Autodesk Inventor part; units mm, degrees
(part 2 of 2)
sketch "Sketch75" plane through (47.5, -21.3496, 62.3406) normal (0, 0.5735764, 0.819152) x (1, 0, 0)
  line L0 (-6.516, 66.3057) -> (-44.6738, 66.3057) construction
  line L1 (-44.6738, 66.3057) -> (-44.6738, 71.3022) construction
  line L2 (-44.6738, 71.3022) -> (-6.516, 71.3022) construction
  line L3 (-6.516, 71.3022) -> (-6.516, 66.3057) construction
  line L4 (-3.768, 77.8286) -> (-3.768, -61.6175) projected
  spline S0 degree 2 poles (-9.2281, 67.8964) (-9.2281, 68.3138) (-8.8897, 68.9857) (-8.6056, 69.1734) knots 0 0 0 1 2 2 2
  spline S1 degree 2 poles (-8.6056, 69.1734) (-8.3735, 69.3191) (-7.8967, 69.4179) (-7.5262, 69.4179) knots 0 0 0 1 2 2 2
  line L5 (-7.5262, 69.4179) -> (-6.8248, 69.4179)
  line L6 (-6.8248, 69.4179) -> (-6.8248, 66.3699)
  line L7 (-6.8248, 66.3699) -> (-7.5188, 66.3699)
  spline S2 degree 2 poles (-7.5188, 66.3699) (-7.9486, 66.3699) (-8.4377, 66.4984) (-8.6106, 66.612) knots 0 0 0 1 2 2 2
  spline S3 degree 2 poles (-8.6106, 66.612) (-8.9045, 66.8071) (-9.2281, 67.4518) (-9.2281, 67.8964) knots 0 0 0 1 2 2 2
  spline S4 degree 2 poles (-8.8057, 67.8915) (-8.8057, 67.5407) (-8.5735, 67.0443) (-8.3438, 66.9035) knots 0 0 0 1 2 2 2
  spline S5 degree 2 poles (-8.3438, 66.9035) (-8.1808, 66.8071) (-7.8128, 66.7207) (-7.5386, 66.7207) knots 0 0 0 1 2 2 2
  line L8 (-7.5386, 66.7207) -> (-7.2298, 66.7207)
  line L9 (-7.2298, 66.7207) -> (-7.2298, 69.0672)
  line L10 (-7.2298, 69.0672) -> (-7.5386, 69.0672)
  spline S6 degree 2 poles (-7.5386, 69.0672) (-7.8078, 69.0672) (-8.2154, 68.9808) (-8.3809, 68.8647) knots 0 0 0 1 2 2 2
  spline S7 degree 2 poles (-8.3809, 68.8647) (-8.5933, 68.7214) (-8.8057, 68.2472) (-8.8057, 67.8915) knots 0 0 0 1 2 2 2
  spline S8 degree 2 poles (-10.7323, 69.4822) (-10.4631, 69.4822) (-10.0629, 69.3414) (-9.9222, 69.2006) knots 0 0 0 1 2 2 2
  spline S9 degree 2 poles (-9.9222, 69.2006) (-9.7616, 69.0425) (-9.6307, 68.5979) (-9.6307, 68.2719) knots 0 0 0 1 2 2 2
  line L11 (-9.6307, 68.2719) -> (-9.6307, 66.3699)
  line L12 (-9.6307, 66.3699) -> (-10.0358, 66.3699)
  line L13 (-10.0358, 66.3699) -> (-10.0358, 68.2719)
  spline S10 degree 2 poles (-10.0358, 68.2719) (-10.0358, 68.4843) (-10.0901, 68.7708) (-10.1667, 68.8869) knots 0 0 0 1 2 2 2
  spline S11 degree 2 poles (-10.1667, 68.8869) (-10.2482, 69.0104) (-10.5298, 69.1364) (-10.7323, 69.1364) knots 0 0 0 1 2 2 2
  spline S12 degree 2 poles (-10.7323, 69.1364) (-10.9225, 69.1364) (-11.2189, 69.0104) (-11.3004, 68.8869) knots 0 0 0 1 2 2 2
  spline S13 degree 2 poles (-11.3004, 68.8869) (-11.377, 68.7708) (-11.4313, 68.4867) (-11.4313, 68.2817) knots 0 0 0 1 2 2 2
  line L14 (-11.4313, 68.2817) -> (-11.4313, 66.3699)
  line L15 (-11.4313, 66.3699) -> (-11.8364, 66.3699)
  line L16 (-11.8364, 66.3699) -> (-11.8364, 68.2719)
  spline S14 degree 2 poles (-11.8364, 68.2719) (-11.8364, 68.5905) (-11.708, 69.045) (-11.545, 69.2006) knots 0 0 0 1 2 2 2
  spline S15 degree 2 poles (-11.545, 69.2006) (-11.3992, 69.3438) (-11.0139, 69.4822) (-10.7323, 69.4822) knots 0 0 0 1 2 2 2
  line L17 (-12.0884, 69.4179) -> (-13.1159, 66.3699)
  line L18 (-13.1159, 66.3699) -> (-13.6148, 66.3699)
  line L19 (-13.6148, 66.3699) -> (-14.6424, 69.4179)
  line L20 (-14.6424, 69.4179) -> (-14.215, 69.4179)
  line L21 (-14.215, 69.4179) -> (-13.9384, 68.5658)
  line L22 (-13.9384, 68.5658) -> (-12.775, 68.5658)
  line L23 (-12.775, 68.5658) -> (-12.4984, 69.4179)
  line L24 (-12.4984, 69.4179) -> (-12.0884, 69.4179)
  line L25 (-13.8272, 68.22) -> (-13.3555, 66.7849)
  line L26 (-13.3555, 66.7849) -> (-12.8862, 68.22)
  line L27 (-12.8862, 68.22) -> (-13.8272, 68.22)
  line L28 (-16.6974, 69.4179) -> (-14.9313, 69.4179)
  line L29 (-14.9313, 69.4179) -> (-14.9313, 66.3699)
  line L30 (-14.9313, 66.3699) -> (-15.3364, 66.3699)
  line L31 (-15.3364, 66.3699) -> (-15.3364, 69.0573)
  line L32 (-15.3364, 69.0573) -> (-16.6974, 69.0573)
  line L33 (-16.6974, 69.0573) -> (-16.6974, 69.4179)
  line L34 (-20.5358, 66.3699) -> (-19.4861, 69.4179)
  line L35 (-19.4861, 69.4179) -> (-19.0489, 69.4179)
  line L36 (-19.0489, 69.4179) -> (-17.9991, 66.3699)
  line L37 (-17.9991, 66.3699) -> (-18.4338, 66.3699)
  line L38 (-18.4338, 66.3699) -> (-19.2786, 68.9017)
  line L39 (-19.2786, 68.9017) -> (-20.1233, 66.3699)
  line L40 (-20.1233, 66.3699) -> (-20.5358, 66.3699)
  line L41 (-21.8894, 69.4179) -> (-20.7087, 69.4179)
  line L42 (-20.7087, 69.4179) -> (-20.7087, 69.1067)
  line L43 (-20.7087, 69.1067) -> (-21.0965, 69.1067)
  line L44 (-21.0965, 69.1067) -> (-21.0965, 66.6812)
  line L45 (-21.0965, 66.6812) -> (-20.7087, 66.6812)
  line L46 (-20.7087, 66.6812) -> (-20.7087, 66.3699)
  line L47 (-20.7087, 66.3699) -> (-21.8894, 66.3699)
  line L48 (-21.8894, 66.3699) -> (-21.8894, 66.6812)
  line L49 (-21.8894, 66.6812) -> (-21.5016, 66.6812)
  line L50 (-21.5016, 66.6812) -> (-21.5016, 69.1067)
  line L51 (-21.5016, 69.1067) -> (-21.8894, 69.1067)
  line L52 (-21.8894, 69.1067) -> (-21.8894, 69.4179)
  spline S16 degree 2 poles (-23.2405, 69.4723) (-22.9095, 69.4723) (-22.4451, 69.334) (-22.2401, 69.2352) knots 0 0 0 1 2 2 2
  line L53 (-22.2401, 69.2352) -> (-22.2401, 68.7263)
  line L54 (-22.2401, 68.7263) -> (-22.2698, 68.7263)
  spline S17 degree 2 poles (-22.2698, 68.7263) (-22.4698, 68.9141) (-22.9762, 69.1215) (-23.2108, 69.1215) knots 0 0 0 1 2 2 2
  spline S18 degree 2 poles (-23.2108, 69.1215) (-23.5468, 69.1215) (-23.8901, 68.8424) (-23.8901, 68.6127) knots 0 0 0 1 2 2 2
  spline S19 degree 2 poles (-23.8901, 68.6127) (-23.8901, 68.4299) (-23.7098, 68.2027) (-23.5147, 68.1459) knots 0 0 0 1 2 2 2
  spline S20 degree 2 poles (-23.5147, 68.1459) (-23.3739, 68.1064) (-23.1392, 68.052) (-22.9638, 68.0076) knots 0 0 0 1 2 2 2
  spline S21 degree 2 poles (-22.9638, 68.0076) (-22.8058, 67.9656) (-22.5563, 67.8396) (-22.46, 67.7383) knots 0 0 0 1 2 2 2
  spline S22 degree 2 poles (-22.46, 67.7383) (-22.3661, 67.6371) (-22.2624, 67.3654) (-22.2624, 67.1875) knots 0 0 0 1 2 2 2
  spline S23 degree 2 poles (-22.2624, 67.1875) (-22.2624, 66.817) (-22.8403, 66.3156) (-23.2874, 66.3156) knots 0 0 0 1 2 2 2
  spline S24 degree 2 poles (-23.2874, 66.3156) (-23.5443, 66.3156) (-23.9988, 66.4169) (-24.1939, 66.5132) knots 0 0 0 1 2 2 2
  line L55 (-24.1939, 66.5132) -> (-24.1939, 66.9973)
  line L56 (-24.1939, 66.9973) -> (-24.1643, 66.9973)
  spline S25 degree 2 poles (-24.1643, 66.9973) (-24.0185, 66.8639) (-23.5641, 66.6663) (-23.3146, 66.6663) knots 0 0 0 1 2 2 2
  spline S26 degree 2 poles (-23.3146, 66.6663) (-23.033, 66.6663) (-22.6847, 66.9306) (-22.6847, 67.1455) knots 0 0 0 1 2 2 2
  spline S27 degree 2 poles (-22.6847, 67.1455) (-22.6847, 67.3382) (-22.8897, 67.5679) (-23.0824, 67.6198) knots 0 0 0 1 2 2 2
  spline S28 degree 2 poles (-23.0824, 67.6198) (-23.2108, 67.6544) (-23.5838, 67.7433) (-23.7073, 67.7803) knots 0 0 0 1 2 2 2
  spline S29 degree 2 poles (-23.7073, 67.7803) (-24.021, 67.8767) (-24.3125, 68.2644) (-24.3125, 68.5485) knots 0 0 0 1 2 2 2
  spline S30 degree 2 poles (-24.3125, 68.5485) (-24.3125, 68.7288) (-24.1667, 69.0746) (-24.0358, 69.1956) knots 0 0 0 1 2 2 2
  spline S31 degree 2 poles (-24.0358, 69.1956) (-23.8901, 69.329) (-23.5196, 69.4723) (-23.2405, 69.4723) knots 0 0 0 1 2 2 2
  line L57 (-25.7871, 69.4179) -> (-24.6064, 69.4179)
  line L58 (-24.6064, 69.4179) -> (-24.6064, 69.1067)
  line L59 (-24.6064, 69.1067) -> (-24.9942, 69.1067)
  line L60 (-24.9942, 69.1067) -> (-24.9942, 66.6812)
  line L61 (-24.9942, 66.6812) -> (-24.6064, 66.6812)
  line L62 (-24.6064, 66.6812) -> (-24.6064, 66.3699)
  line L63 (-24.6064, 66.3699) -> (-25.7871, 66.3699)
  line L64 (-25.7871, 66.3699) -> (-25.7871, 66.6812)
  line L65 (-25.7871, 66.6812) -> (-25.3993, 66.6812)
  line L66 (-25.3993, 66.6812) -> (-25.3993, 69.1067)
  line L67 (-25.3993, 69.1067) -> (-25.7871, 69.1067)
  line L68 (-25.7871, 69.1067) -> (-25.7871, 69.4179)
  spline S32 degree 2 poles (-28.4448, 66.7182) (-28.6177, 66.9208) (-28.8104, 67.5136) (-28.8104, 67.8939) knots 0 0 0 1 2 2 2
  spline S33 degree 2 poles (-28.8104, 67.8939) (-28.8104, 68.2644) (-28.6226, 68.8647) (-28.4448, 69.0672) knots 0 0 0 1 2 2 2
  spline S34 degree 2 poles (-28.4448, 69.0672) (-28.2571, 69.2796) (-27.7606, 69.4822) (-27.4617, 69.4822) knots 0 0 0 1 2 2 2
  spline S35 degree 2 poles (-27.4617, 69.4822) (-27.153, 69.4822) (-26.659, 69.2722) (-26.4787, 69.0672) knots 0 0 0 1 2 2 2
  spline S36 degree 2 poles (-26.4787, 69.0672) (-26.3033, 68.8647) (-26.1156, 68.2694) (-26.1156, 67.8939) knots 0 0 0 1 2 2 2
  spline S37 degree 2 poles (-26.1156, 67.8939) (-26.1156, 67.5111) (-26.3058, 66.9282) (-26.4811, 66.7182) knots 0 0 0 1 2 2 2
  spline S38 degree 2 poles (-26.4811, 66.7182) (-26.659, 66.5157) (-27.1555, 66.3057) (-27.4617, 66.3057) knots 0 0 0 1 2 2 2
  spline S39 degree 2 poles (-27.4617, 66.3057) (-27.773, 66.3057) (-28.2719, 66.5231) (-28.4448, 66.7182) knots 0 0 0 1 2 2 2
  spline S40 degree 2 poles (-28.388, 67.8939) (-28.388, 67.5926) (-28.2571, 67.1258) (-28.1385, 66.9726) knots 0 0 0 1 2 2 2
  spline S41 degree 2 poles (-28.1385, 66.9726) (-28.0175, 66.8145) (-27.6766, 66.6565) (-27.4642, 66.6565) knots 0 0 0 1 2 2 2
  spline S42 degree 2 poles (-27.4642, 66.6565) (-27.2444, 66.6565) (-26.9134, 66.8096) (-26.7874, 66.9726) knots 0 0 0 1 2 2 2
  spline S43 degree 2 poles (-26.7874, 66.9726) (-26.6664, 67.1282) (-26.538, 67.5975) (-26.538, 67.8939) knots 0 0 0 1 2 2 2
  spline S44 degree 2 poles (-26.538, 67.8939) (-26.538, 68.4942) (-27.0418, 69.1314) (-27.4642, 69.1314) knots 0 0 0 1 2 2 2
  spline S45 degree 2 poles (-27.4642, 69.1314) (-27.8866, 69.1314) (-28.388, 68.4942) (-28.388, 67.8939) knots 0 0 0 1 2 2 2
  line L69 (-31.436, 69.4179) -> (-30.9815, 69.4179)
  line L70 (-30.9815, 69.4179) -> (-29.6329, 66.7898)
  line L71 (-29.6329, 66.7898) -> (-29.6329, 69.4179)
  line L72 (-29.6329, 69.4179) -> (-29.255, 69.4179)
  line L73 (-29.255, 69.4179) -> (-29.255, 66.3699)
  line L74 (-29.255, 66.3699) -> (-29.8305, 66.3699)
  line L75 (-29.8305, 66.3699) -> (-31.0581, 68.7832)
  line L76 (-31.0581, 68.7832) -> (-31.0581, 66.3699)
  line L77 (-31.0581, 66.3699) -> (-31.436, 66.3699)
  line L78 (-31.436, 66.3699) -> (-31.436, 69.4179)
  line L79 (-35.1287, 69.4179) -> (-33.3626, 69.4179)
  line L80 (-33.3626, 69.4179) -> (-33.3626, 66.3699)
  line L81 (-33.3626, 66.3699) -> (-33.7677, 66.3699)
  line L82 (-33.7677, 66.3699) -> (-33.7677, 69.0573)
  line L83 (-33.7677, 69.0573) -> (-35.1287, 69.0573)
  line L84 (-35.1287, 69.0573) -> (-35.1287, 69.4179)
  line L85 (-36.5094, 69.4179) -> (-35.3287, 69.4179)
  line L86 (-35.3287, 69.4179) -> (-35.3287, 69.1067)
  line L87 (-35.3287, 69.1067) -> (-35.7165, 69.1067)
  line L88 (-35.7165, 69.1067) -> (-35.7165, 66.6812)
  line L89 (-35.7165, 66.6812) -> (-35.3287, 66.6812)
  line L90 (-35.3287, 66.6812) -> (-35.3287, 66.3699)
  line L91 (-35.3287, 66.3699) -> (-36.5094, 66.3699)
  line L92 (-36.5094, 66.3699) -> (-36.5094, 66.6812)
  line L93 (-36.5094, 66.6812) -> (-36.1216, 66.6812)
  line L94 (-36.1216, 66.6812) -> (-36.1216, 69.1067)
  line L95 (-36.1216, 69.1067) -> (-36.5094, 69.1067)
  line L96 (-36.5094, 69.1067) -> (-36.5094, 69.4179)
  spline S46 degree 2 poles (-39.4141, 67.8964) (-39.4141, 68.3138) (-39.0758, 68.9857) (-38.7917, 69.1734) knots 0 0 0 1 2 2 2
  spline S47 degree 2 poles (-38.7917, 69.1734) (-38.5595, 69.3191) (-38.0828, 69.4179) (-37.7123, 69.4179) knots 0 0 0 1 2 2 2
  line L97 (-37.7123, 69.4179) -> (-37.0108, 69.4179)
  line L98 (-37.0108, 69.4179) -> (-37.0108, 66.3699)
  line L99 (-37.0108, 66.3699) -> (-37.7049, 66.3699)
  spline S48 degree 2 poles (-37.7049, 66.3699) (-38.1347, 66.3699) (-38.6237, 66.4984) (-38.7966, 66.612) knots 0 0 0 1 2 2 2
  spline S49 degree 2 poles (-38.7966, 66.612) (-39.0906, 66.8071) (-39.4141, 67.4518) (-39.4141, 67.8964) knots 0 0 0 1 2 2 2
  spline S50 degree 2 poles (-38.9918, 67.8915) (-38.9918, 67.5407) (-38.7596, 67.0443) (-38.5299, 66.9035) knots 0 0 0 1 2 2 2
  spline S51 degree 2 poles (-38.5299, 66.9035) (-38.3669, 66.8071) (-37.9988, 66.7207) (-37.7247, 66.7207) knots 0 0 0 1 2 2 2
  line L100 (-37.7247, 66.7207) -> (-37.4159, 66.7207)
  line L101 (-37.4159, 66.7207) -> (-37.4159, 69.0672)
  line L102 (-37.4159, 69.0672) -> (-37.7247, 69.0672)
  spline S52 degree 2 poles (-37.7247, 69.0672) (-37.9939, 69.0672) (-38.4014, 68.9808) (-38.5669, 68.8647) knots 0 0 0 1 2 2 2
  spline S53 degree 2 poles (-38.5669, 68.8647) (-38.7794, 68.7214) (-38.9918, 68.2472) (-38.9918, 67.8915) knots 0 0 0 1 2 2 2
  line L103 (-8.6526, 71.8454) -> (-7.3336, 74.4364)
  line L104 (-7.3336, 74.4364) -> (-6.8989, 74.4364)
  line L105 (-6.8989, 74.4364) -> (-8.2919, 71.7465)
  line L106 (-8.2919, 71.7465) -> (-6.7185, 71.7465)
  line L107 (-6.7185, 71.7465) -> (-6.7185, 71.3884)
  line L108 (-6.7185, 71.3884) -> (-8.6526, 71.3884)
  line L109 (-8.6526, 71.3884) -> (-8.6526, 71.8454)
  line L110 (-9.6801, 74.4364) -> (-9.191, 74.4364)
  line L111 (-9.191, 74.4364) -> (-9.191, 73.8535)
  line L112 (-9.191, 73.8535) -> (-9.6801, 73.8535)
  line L113 (-9.6801, 73.8535) -> (-9.6801, 74.4364)
  line L114 (-12.1748, 74.4364) -> (-10.2951, 74.4364)
  line L115 (-10.2951, 74.4364) -> (-10.2951, 74.0041)
  spline S54 degree 2 poles (-10.2951, 74.0041) (-10.4977, 73.814) (-10.8583, 73.4607) (-11.0312, 73.2705) knots 0 0 0 1 2 2 2
  spline S55 degree 2 poles (-11.0312, 73.2705) (-11.3795, 72.8877) (-11.6339, 72.4283) (-11.6339, 72.1837) knots 0 0 0 1 2 2 2
  spline S56 degree 2 poles (-11.6339, 72.1837) (-11.6339, 72.0553) (-11.5548, 71.8626) (-11.4832, 71.8009) knots 0 0 0 1 2 2 2
  spline S57 degree 2 poles (-11.4832, 71.8009) (-11.4116, 71.7391) (-11.2239, 71.6774) (-11.1102, 71.6774) knots 0 0 0 1 2 2 2
  spline S58 degree 2 poles (-11.1102, 71.6774) (-11.0015, 71.6774) (-10.7792, 71.7317) (-10.678, 71.7737) knots 0 0 0 1 2 2 2
  spline S59 degree 2 poles (-10.678, 71.7737) (-10.5915, 71.8083) (-10.431, 71.9071) (-10.3816, 71.9417) knots 0 0 0 1 2 2 2
  line L116 (-10.3816, 71.9417) -> (-10.3593, 71.9417)
  line L117 (-10.3593, 71.9417) -> (-10.3593, 71.507)
  spline S60 degree 2 poles (-10.3593, 71.507) (-10.4853, 71.4452) (-10.9373, 71.3242) (-11.1399, 71.3242) knots 0 0 0 1 2 2 2
  spline S61 degree 2 poles (-11.1399, 71.3242) (-11.5672, 71.3242) (-12.0488, 71.7762) (-12.0488, 72.1615) knots 0 0 0 1 2 2 2
  spline S62 degree 2 poles (-12.0488, 72.1615) (-12.0488, 72.3418) (-11.9649, 72.6432) (-11.8908, 72.7716) knots 0 0 0 1 2 2 2
  spline S63 degree 2 poles (-11.8908, 72.7716) (-11.8167, 72.905) (-11.6018, 73.1668) (-11.4832, 73.2928) knots 0 0 0 1 2 2 2
  spline S64 degree 2 poles (-11.4832, 73.2928) (-11.2905, 73.5027) (-10.8188, 73.9523) (-10.678, 74.0832) knots 0 0 0 1 2 2 2
  line L118 (-10.678, 74.0832) -> (-12.1748, 74.0832)
  line L119 (-12.1748, 74.0832) -> (-12.1748, 74.4364)
  spline S65 degree 2 poles (-13.4049, 71.6774) (-13.2937, 71.6774) (-13.0739, 71.7317) (-12.9677, 71.7737) knots 0 0 0 1 2 2 2
  spline S66 degree 2 poles (-12.9677, 71.7737) (-12.8689, 71.8157) (-12.7232, 71.9046) (-12.6663, 71.9442) knots 0 0 0 1 2 2 2
  line L120 (-12.6663, 71.9442) -> (-12.6416, 71.9442)
  line L121 (-12.6416, 71.9442) -> (-12.6416, 71.5119)
  spline S67 degree 2 poles (-12.6416, 71.5119) (-12.775, 71.4403) (-13.232, 71.3242) (-13.437, 71.3242) knots 0 0 0 1 2 2 2
  spline S68 degree 2 poles (-13.437, 71.3242) (-13.6445, 71.3242) (-13.9532, 71.4082) (-14.0792, 71.4971) knots 0 0 0 1 2 2 2
  spline S69 degree 2 poles (-14.0792, 71.4971) (-14.2126, 71.5934) (-14.3509, 71.8725) (-14.3509, 72.0602) knots 0 0 0 1 2 2 2
  spline S70 degree 2 poles (-14.3509, 72.0602) (-14.3509, 72.3122) (-14.0199, 72.6926) (-13.7877, 72.742) knots 0 0 0 1 2 2 2
  line L122 (-13.7877, 72.742) -> (-13.7877, 72.7716)
  spline S71 degree 2 poles (-13.7877, 72.7716) (-13.8841, 72.7914) (-14.1039, 72.8803) (-14.1978, 72.9692) knots 0 0 0 1 2 2 2
  spline S72 degree 2 poles (-14.1978, 72.9692) (-14.2916, 73.0557) (-14.4102, 73.3323) (-14.4102, 73.5324) knots 0 0 0 1 2 2 2
  spline S73 degree 2 poles (-14.4102, 73.5324) (-14.4102, 73.7374) (-14.2694, 74.0857) (-14.1409, 74.219) knots 0 0 0 1 2 2 2
  spline S74 degree 2 poles (-14.1409, 74.219) (-14.0076, 74.3574) (-13.6296, 74.5006) (-13.3901, 74.5006) knots 0 0 0 1 2 2 2
  spline S75 degree 2 poles (-13.3901, 74.5006) (-13.1603, 74.5006) (-12.7108, 74.3895) (-12.5577, 74.3129) knots 0 0 0 1 2 2 2
  line L123 (-12.5577, 74.3129) -> (-12.5577, 73.8806)
  line L124 (-12.5577, 73.8806) -> (-12.5873, 73.8806)
  spline S76 degree 2 poles (-12.5873, 73.8806) (-12.7157, 73.9745) (-13.1505, 74.1474) (-13.3654, 74.1474) knots 0 0 0 1 2 2 2
  spline S77 degree 2 poles (-13.3654, 74.1474) (-13.4913, 74.1474) (-13.7433, 74.0684) (-13.8272, 73.977) knots 0 0 0 1 2 2 2
  spline S78 degree 2 poles (-13.8272, 73.977) (-13.9088, 73.8856) (-13.9952, 73.6682) (-13.9952, 73.5027) knots 0 0 0 1 2 2 2
  spline S79 degree 2 poles (-13.9952, 73.5027) (-13.9952, 73.3372) (-13.8989, 73.1223) (-13.8124, 73.0606) knots 0 0 0 1 2 2 2
  spline S80 degree 2 poles (-13.8124, 73.0606) (-13.726, 72.9988) (-13.4913, 72.9519) (-13.353, 72.9519) knots 0 0 0 1 2 2 2
  line L125 (-13.353, 72.9519) -> (-13.1801, 72.9519)
  line L126 (-13.1801, 72.9519) -> (-13.1801, 72.6135)
  line L127 (-13.1801, 72.6135) -> (-13.316, 72.6135)
  spline S81 degree 2 poles (-13.316, 72.6135) (-13.5901, 72.6135) (-13.9359, 72.3517) (-13.9359, 72.1022) knots 0 0 0 1 2 2 2
  spline S82 degree 2 poles (-13.9359, 72.1022) (-13.9359, 71.9861) (-13.847, 71.8207) (-13.7754, 71.7712) knots 0 0 0 1 2 2 2
  spline S83 degree 2 poles (-13.7754, 71.7712) (-13.6988, 71.7194) (-13.5111, 71.6774) (-13.4049, 71.6774) knots 0 0 0 1 2 2 2
  line L128 (-15.5241, 74.4364) -> (-15.0351, 74.4364)
  line L129 (-15.0351, 74.4364) -> (-15.0351, 73.8535)
  line L130 (-15.0351, 73.8535) -> (-15.5241, 73.8535)
  line L131 (-15.5241, 73.8535) -> (-15.5241, 74.4364)
  line L132 (-18.0189, 74.4364) -> (-16.1392, 74.4364)
  line L133 (-16.1392, 74.4364) -> (-16.1392, 74.0041)
  spline S84 degree 2 poles (-16.1392, 74.0041) (-16.3417, 73.814) (-16.7023, 73.4607) (-16.8752, 73.2705) knots 0 0 0 1 2 2 2
  spline S85 degree 2 poles (-16.8752, 73.2705) (-17.2235, 72.8877) (-17.4779, 72.4283) (-17.4779, 72.1837) knots 0 0 0 1 2 2 2
  spline S86 degree 2 poles (-17.4779, 72.1837) (-17.4779, 72.0553) (-17.3989, 71.8626) (-17.3273, 71.8009) knots 0 0 0 1 2 2 2
  spline S87 degree 2 poles (-17.3273, 71.8009) (-17.2556, 71.7391) (-17.0679, 71.6774) (-16.9543, 71.6774) knots 0 0 0 1 2 2 2
  spline S88 degree 2 poles (-16.9543, 71.6774) (-16.8456, 71.6774) (-16.6233, 71.7317) (-16.522, 71.7737) knots 0 0 0 1 2 2 2
  spline S89 degree 2 poles (-16.522, 71.7737) (-16.4356, 71.8083) (-16.275, 71.9071) (-16.2256, 71.9417) knots 0 0 0 1 2 2 2
  line L134 (-16.2256, 71.9417) -> (-16.2034, 71.9417)
  line L135 (-16.2034, 71.9417) -> (-16.2034, 71.507)
  spline S90 degree 2 poles (-16.2034, 71.507) (-16.3294, 71.4452) (-16.7814, 71.3242) (-16.9839, 71.3242) knots 0 0 0 1 2 2 2
  spline S91 degree 2 poles (-16.9839, 71.3242) (-17.4112, 71.3242) (-17.8929, 71.7762) (-17.8929, 72.1615) knots 0 0 0 1 2 2 2
  spline S92 degree 2 poles (-17.8929, 72.1615) (-17.8929, 72.3418) (-17.8089, 72.6432) (-17.7348, 72.7716) knots 0 0 0 1 2 2 2
  spline S93 degree 2 poles (-17.7348, 72.7716) (-17.6607, 72.905) (-17.4458, 73.1668) (-17.3273, 73.2928) knots 0 0 0 1 2 2 2
  spline S94 degree 2 poles (-17.3273, 73.2928) (-17.1346, 73.5027) (-16.6628, 73.9523) (-16.522, 74.0832) knots 0 0 0 1 2 2 2
  line L136 (-16.522, 74.0832) -> (-18.0189, 74.0832)
  line L137 (-18.0189, 74.0832) -> (-18.0189, 74.4364)
  spline S95 degree 2 poles (-20.274, 73.4682) (-20.274, 73.688) (-20.1332, 74.0634) (-20.0048, 74.2017) knots 0 0 0 1 2 2 2
  spline S96 degree 2 poles (-20.0048, 74.2017) (-19.8763, 74.3401) (-19.4935, 74.5006) (-19.2563, 74.5006) knots 0 0 0 1 2 2 2
  spline S97 degree 2 poles (-19.2563, 74.5006) (-19.039, 74.5006) (-18.6141, 74.4043) (-18.4585, 74.3277) knots 0 0 0 1 2 2 2
  line L138 (-18.4585, 74.3277) -> (-18.4585, 73.8955)
  line L139 (-18.4585, 73.8955) -> (-18.4882, 73.8955)
  spline S98 degree 2 poles (-18.4882, 73.8955) (-18.5351, 73.93) (-18.7105, 74.019) (-18.8167, 74.0585) knots 0 0 0 1 2 2 2
  spline S99 degree 2 poles (-18.8167, 74.0585) (-18.9377, 74.1005) (-19.1378, 74.1474) (-19.2638, 74.1474) knots 0 0 0 1 2 2 2
  spline S100 degree 2 poles (-19.2638, 74.1474) (-19.3873, 74.1474) (-19.6194, 74.0585) (-19.7034, 73.9622) knots 0 0 0 1 2 2 2
  spline S101 degree 2 poles (-19.7034, 73.9622) (-19.78, 73.8708) (-19.859, 73.6287) (-19.859, 73.4657) knots 0 0 0 1 2 2 2
  spline S102 degree 2 poles (-19.859, 73.4657) (-19.859, 73.3027) (-19.7701, 73.0952) (-19.6861, 73.026) knots 0 0 0 1 2 2 2
  spline S103 degree 2 poles (-19.6861, 73.026) (-19.5997, 72.9494) (-19.3428, 72.8852) (-19.1872, 72.8852) knots 0 0 0 1 2 2 2
  spline S104 degree 2 poles (-19.1872, 72.8852) (-19.0192, 72.8852) (-18.6858, 72.9371) (-18.5845, 72.9593) knots 0 0 0 1 2 2 2
  line L140 (-18.5845, 72.9593) -> (-18.5845, 71.3884)
  line L141 (-18.5845, 71.3884) -> (-20.2567, 71.3884)
  line L142 (-20.2567, 71.3884) -> (-20.2567, 71.7465)
  line L143 (-20.2567, 71.7465) -> (-18.9772, 71.7465)
  line L144 (-18.9772, 71.7465) -> (-18.9772, 72.5592)
  spline S105 degree 2 poles (-18.9772, 72.5592) (-19.0513, 72.5493) (-19.1946, 72.5419) (-19.2539, 72.5419) knots 0 0 0 1 2 2 2
  spline S106 degree 2 poles (-19.2539, 72.5419) (-19.4885, 72.5419) (-19.8121, 72.6185) (-19.9603, 72.7321) knots 0 0 0 1 2 2 2
  spline S107 degree 2 poles (-19.9603, 72.7321) (-20.111, 72.8457) (-20.274, 73.1915) (-20.274, 73.4682) knots 0 0 0 1 2 2 2
  point P0 (-3.768, -60.8007)
  point P1 (-6.516, 68.804)
  dimension "d262" = 2.748
  constraints: 1 midpoint, 2 other
  measures "d262" distance from line of point (-6.516, 68.804) L4
extrude "Extrusion64" add sketch "Sketch75" along normal blind 1
sketch "Sketch76" plane through (43.732, -87.3592, 75.4961) normal (0, 0.819152, -0.5735764) x (1, 0, 0)
  line L0 (0, 0) -> (6, 0) projected
  line L1 (6, 46.3654) -> (6, 0) projected
  line L2 (6, 0) -> (6, 5)
  line L3 (6, 5) -> (2.5, 5)
  line L4 (2.5, 5) -> (5.3868, 0)
  line L5 (6, 0) -> (5.3868, 0)
  line L6 (-98.464, 0) -> (-98.464, 5)
  line L7 (-98.464, 13.3654) -> (-98.464, -7.5921) projected
  line L8 (-98.464, 5) -> (-94.964, 5)
  line L9 (-94.964, 5) -> (-97.8508, 0)
  line L10 (6, 0) -> (6, -0.5045)
  line L11 (6, 0) -> (6, -21.0852) projected
  line L12 (5.6934, -0.5045) -> (5.3868, 0)
  line L13 (5.6934, -0.5045) -> (6, -0.5045)
  line L14 (6, 0.2313) -> (6, -0.6163)
  line L15 (6, -0.6163) -> (5.7513, -0.6163)
  line L16 (5.7513, -0.6163) -> (5.3674, 0.0335)
  line L17 (-98.464, 0.2313) -> (-98.464, -0.6163)
  line L18 (-98.464, -0.6163) -> (-98.0058, -0.6163)
  line L19 (-98.0058, -0.6163) -> (-97.8508, 0)
  point P0 (-43.732, 11.7356)
  point P1 (-98.464, 0)
  dimension "d266" = 3.5
  dimension "d268" = 5
  dimension "d269" = 3.5
  dimension "d270" = 60
  constraints: 32 end point, 9 point on line, 3 horizontal, 3 perpendicular
  measures "d266" distance of L2.end L3.end
  measures "d268" distance of L6.start L6.end
  measures "d269" distance of L6.end L8.end
  measures "d270" angle of L8 L9
extrude "Extrusion65" add sketch "Sketch76" along normal blind 100.764 contours L4 L3 L1 L0 | L6 L8 L9 L19 L18 L7
body "Solid1"
